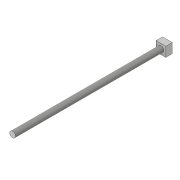
# Autodesk Inventor part: 23CM NUT
Saved by Autodesk Inventor 2019 (Build 230136000, 136)
## iProperties
Created: 2019-10-07
Part Number: 23CM NUT
Material: Generic
Document SubType Name: Modeling
Designer: Admin
Density: 1 g/cm^3
Appearance: Default
Author: Admin
Autodesk Inventor part; units mm, degrees
ref_plane "YZ Plane" through (0, 0, 0) normal (1, 0, 0) x (0, 1, 0)
ref_plane "XZ Plane" through (0, 0, 0) normal (0, 1, 0) x (-1, 0, 0)
sketch "Sketch1" plane through (0, 0, 0) normal (0, 0, 1) x (1, 0, 0)
  line L0 (0, 0) -> (15, 0)
  line L1 (15, 0) -> (15, 15)
  line L2 (15, 15) -> (0, 15)
  line L3 (0, 15) -> (0, 0)
  dimension "d0" = 15
  dimension "d1" = 15
  constraints: 8 end point, 2 parallel, 1 horizontal, 1 perpendicular
  measures "d0" distance of L2.end L1.end
  measures "d1" distance of L1.end L0.end
extrude "Extrusion1" add sketch "Sketch1" along normal blind 10
sketch "Sketch2" plane through (0, 0, 10) normal (0, 0, 1) x (1, 0, 0)
  line L0 (15, 15) -> (0, 15) projected
  line L1 (0, 15) -> (7.5, 15)
  line L2 (7.5, 15) -> (7.5, 0.4087)
  line L3 (0, 15) -> (0, 0) projected
  line L4 (0, 7.7044) -> (14.7572, 7.5)
  circle A0 centre (7.5, 7.7044) radius 4.5
  dimension "d9" = 9
  constraints: 6 end point, 2 midpoint, 1 centre point, 1 point on line
  measures "d9" diameter of A0
extrude "Extrusion2" add sketch "Sketch2" along normal blind 230 contours A0 L4 L2 | L2 L4 A0 | L4 A0 L2 | L2 A0 L4
thread "Thread1" size "M11x1.5" class "6g" standard "ANSI Metric M Profile" full length
thread "Thread2" size "M9x1.25" class "6g" standard "ANSI Metric M Profile" full length
sketch "Sketch3" plane through (0, 0, 0) normal (1, 0, 0) x (0, 1, 0)
  point P0 (0, 0)
ref_plane "Work Plane1" through (7.5, 7.7044, 240) normal (0, 0, 1) x (1, 0, 0)
sketch "Sketch4" plane through (7.5, 7.7044, 240) normal (0, 0, 1) x (1, 0, 0)
  point P0 (-7.5, -7.7044)
extrude "Extrusion3" [suppressed]
body "Solid1"
